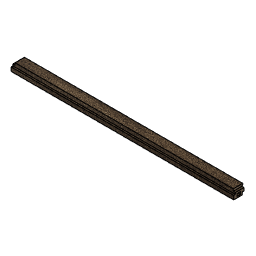
Apron_Long (Autodesk Fusion 360 design; units mm, degrees)
Autodesk Fusion 360 part; units mm, degrees
note: some values were not read from the file. Chosen so that the rebuilt part matches the saved one: where a step ends.
sketch "Sketch1" plane through (0, 0, 0) normal (0, 0, 1) x (1, 0, 0)
  line L0 (-825.5, 41.275) -> (825.5, 41.275)
  line L1 (825.5, 41.275) -> (825.5, -41.275)
  line L2 (825.5, -41.275) -> (-825.5, -41.275)
  line L3 (-825.5, -41.275) -> (-825.5, 41.275)
  line L4 (-825.5, 41.275) -> (825.5, -41.275) construction
  line L5 (825.5, 41.275) -> (-825.5, -41.275) construction
  dimension "d1" = 1651
  dimension "d2" = 82.55
  constraint horizontal L0
  constraint perpendicular L0 L1
  constraint parallel L0 L2
  constraint parallel L1 L3
  constraint coincident L4 origin
  constraint coincident L5 origin
  measures "d1" distance of L1.end L2.end
  measures "d2" distance of L0.end L1.end
extrude "Extrude1" add sketch "Sketch1" along normal blind 57.15
sketch "Sketch8" plane through (825.5, 0, 0) normal (1, 0, 0) x (0, 1, 0)
  line L0 (-41.275, 0) -> (41.275, 0)
  line L1 (41.275, 0) -> (41.275, 57.15)
  line L2 (41.275, 57.15) -> (-41.275, 57.15)
  line L3 (-41.275, 57.15) -> (-41.275, 0)
  line L4 (-41.275, 57.15) -> (-41.275, 28.575)
  line L5 (-41.275, 28.575) -> (-28.575, 28.575)
  line L6 (-28.575, 28.575) -> (-28.575, 57.15)
  line L7 (-28.575, 57.15) -> (-41.275, 57.15)
  line L8 (41.275, 0) -> (22.225, 0)
  line L9 (22.225, 0) -> (22.225, 19.05)
  line L10 (22.225, 19.05) -> (34.925, 19.05)
  line L11 (34.925, 19.05) -> (34.925, 44.45)
  line L12 (34.925, 44.45) -> (41.275, 44.45)
  line L13 (41.275, 0) -> (41.275, 44.45)
  dimension "d27" = 12.7
  dimension "d30" = 19.05
  dimension "d31" = 12.7
  dimension "d32" = 12.7
  dimension "d33" = 19.05
  constraint coincident L2.end L3.start
  constraint midpoint L3 L4.end
  constraint perpendicular L4 L5
  constraint coincident L2 L6.end
  constraint perpendicular L2 L6
  constraint coincident L0.end L1.start
  constraint perpendicular L1 L8
  constraint perpendicular L8 L9
  constraint perpendicular L9 L10
  constraint perpendicular L10 L11
  constraint coincident L1 L12.end
  constraint perpendicular L1 L12
  measures "d27" distance of L4.end L5.end
  measures "d30" distance of L0.end L8.end
  measures "d31" distance of L9.end L10.end
  measures "d32" distance of L2 L12
  measures "d33" distance of L8 L10
extrude "Extrude8" cut sketch "Sketch8" along normal up to far side of body 1 contours L0 L1 L8 L9 L10 L11 L12 L13 | L2 L3 L4 L5 L6 L7
sketch "Sketch12" plane through (0, 0, 57.15) normal (0, 0, -1) x (1, 0, 0)
  line L0 (-825.5, -22.225) -> (-825.5, -34.925)
  line L1 (-825.5, -34.925) -> (825.5, -34.925)
  line L2 (825.5, -34.925) -> (825.5, -22.225)
  line L3 (825.5, -22.225) -> (-825.5, -22.225)
  line L4 (0, -34.925) -> (-30.1625, -34.925)
  line L5 (0, -34.925) -> (30.1625, -34.925)
  line L6 (0, -34.925) -> (0, -22.225) construction
  arc A0 (30.1625, -34.925) -> (-30.1625, -34.925) centre (0, -64.393) ccw
  arc A1 (-579.4375, -34.925) -> (-639.7625, -34.925) centre (-609.6, -64.393) ccw
  line L7 (-609.6, -34.925) -> (-579.4375, -34.925)
  line L8 (-609.6, -34.925) -> (-609.6, -22.225) construction
  line L9 (-609.6, -34.925) -> (-639.7625, -34.925)
  arc A2 (-274.6375, -34.925) -> (-334.9625, -34.925) centre (-304.8, -64.393) ccw
  line L10 (-304.8, -34.925) -> (-274.6375, -34.925)
  line L11 (-304.8, -34.925) -> (-304.8, -22.225) construction
  line L12 (-304.8, -34.925) -> (-334.9625, -34.925)
  arc A3 (334.9625, -34.925) -> (274.6375, -34.925) centre (304.8, -64.393) ccw
  line L13 (304.8, -34.925) -> (334.9625, -34.925)
  line L14 (304.8, -34.925) -> (304.8, -22.225) construction
  line L15 (304.8, -34.925) -> (274.6375, -34.925)
  arc A4 (639.7625, -34.925) -> (579.4375, -34.925) centre (609.6, -64.393) ccw
  line L16 (609.6, -34.925) -> (639.7625, -34.925)
  line L17 (609.6, -34.925) -> (609.6, -22.225) construction
  line L18 (609.6, -34.925) -> (579.4375, -34.925)
  line L19 (-825.5, 28.575) -> (825.5, 28.575)
  line L20 (825.5, 28.575) -> (825.5, -41.275)
  line L21 (825.5, -41.275) -> (-825.5, -41.275)
  line L22 (-825.5, -41.275) -> (-825.5, 28.575)
  dimension "d62" = 60.325
  dimension "d63" = 12.7
  dimension "d66" = 304.8
  dimension "d67" = 0
  constraint midpoint L1 L4.start
  constraint coincident L1 L4.end
  constraint parallel L1 L4
  constraint coincident L1 L5.end
  constraint parallel L1 L5
  constraint equal L4 L5
  constraint perpendicular L5 L6
  constraint coincident L6.end A0
  measures "d62" distance of L4.end L5.end
  measures "d63" distance of L4.start L6.end
extrude "Extrude12" cut sketch "Sketch12" along normal blind 3.7703 from surface at 28.575 contours L1 A1 L7 L9 | L1 A2 L10 L12 | L1 L4 L5 A0 | L1 A3 L13 L15 | L1 A4 L16 L18
sketch "Sketch11" plane through (0, 41.275, 0) normal (0, 1, 0) x (-1, 0, 0)
  line L0 (-825.5, 44.45) -> (825.5, 44.45)
  line L1 (825.5, 44.45) -> (825.5, 57.15)
  line L2 (825.5, 57.15) -> (-825.5, 57.15)
  line L3 (-825.5, 57.15) -> (-825.5, 44.45)
  line L4 (-825.5, 57.15) -> (-809.625, 57.15)
  line L5 (-809.625, 57.15) -> (-809.625, 41.275)
  line L6 (-809.625, 41.275) -> (-825.5, 41.275)
  line L7 (-825.5, 41.275) -> (-825.5, 57.15)
  line L8 (825.5, 57.15) -> (809.625, 57.15)
  line L9 (809.625, 57.15) -> (809.625, 41.275)
  line L10 (809.625, 41.275) -> (825.5, 41.275)
  line L11 (825.5, 41.275) -> (825.5, 57.15)
  dimension "d53" = 15.875
  dimension "d54" = 15.875
  dimension "d55" = 15.875
  dimension "d56" = 15.875
  constraint horizontal L4
  constraint vertical L5
  constraint horizontal L6
  constraint vertical L7
  constraint coincident L2.end L3.start
  constraint horizontal L8
  constraint vertical L9
  constraint horizontal L10
  constraint vertical L11
  constraint coincident L1.end L2.start
  measures "d53" distance of L2.end L4.end
  measures "d54" distance of L2.end L6.end
  measures "d55" distance of L1.end L8.end
  measures "d56" distance of L1.end L10.end
extrude "Extrude11" cut sketch "Sketch11" against normal blind 82.55 contours L0 L2 L3 L4 L5 L7 | L0 L5 L6 L7 | L0 L1 L2 L8 L9 L11 | L0 L9 L10 L11
sketch "Sketch13" plane through (825.5, 0, 0) normal (1, 0, 0) x (0, 1, 0)
  line L0 (34.925, 41.275) -> (-28.575, 41.275)
  line L1 (-28.575, 41.275) -> (-28.575, 28.575)
  line L2 (-28.575, 28.575) -> (-41.275, 28.575)
  line L3 (-41.275, 28.575) -> (-41.275, 0)
  line L4 (-41.275, 0) -> (22.225, 0)
  line L5 (22.225, 0) -> (22.225, 19.05)
  line L6 (22.225, 19.05) -> (34.925, 19.05)
  line L7 (34.925, 19.05) -> (34.925, 41.275)
  line L8 (0, 0) -> (-3.175, 0) construction
  line L9 (-3.175, 0) -> (-3.175, 19.05) construction
  line L10 (9.525, 9.525) -> (-15.875, 9.525)
  line L11 (-15.875, 9.525) -> (-15.875, 28.575)
  line L12 (-15.875, 28.575) -> (9.525, 28.575)
  line L13 (9.525, 28.575) -> (9.525, 9.525)
  line L14 (9.525, 9.525) -> (-15.875, 28.575) construction
  line L15 (-15.875, 9.525) -> (9.525, 28.575) construction
  point P0 (-3.175, 19.05)
  dimension "d71" = 3.175
  dimension "d72" = 19.05
  dimension "d73" = 25.4
  dimension "d74" = 19.05
  constraint coincident L8.start origin
  constraint horizontal L8
  constraint perpendicular L8 L9
  constraint horizontal L10
  constraint perpendicular L10 L11
  constraint parallel L10 L12
  constraint parallel L11 L13
  constraint coincident L14 P0
  constraint coincident L15 P0
  constraint coincident P0 L9.end
  measures "d71" distance of L8.start L8.end
  measures "d72" distance of L8.end P0
  measures "d73" distance of L11.end L12.end
  measures "d74" distance of L10.end L11.end
extrude "Extrude13" cut sketch "Sketch13" against normal blind 38.1 contours L10 L11 L12 L13
extrude "Extrude14" cut sketch "Sketch13" along normal blind 38.1 from surface at -1651 contours L10 L11 L12 L13
equation "d62 = 2 in + ( 3 / 8 ) * 1 in"
equation "d69 = ( 19 / 128 ) * 1 in"
